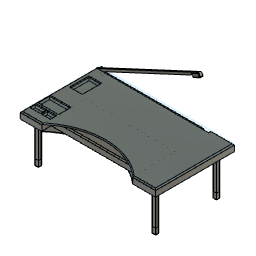
study pad (1) (Autodesk Fusion 360 design; units mm, degrees)
Autodesk Fusion 360 part; units mm, degrees
sketch "Sketch1" plane through (0, 0, 0) normal (0, 0, 1) x (1, 0, 0)
  line L0 (30, -17.5) -> (-30, -17.5)
  line L1 (-30, -17.5) -> (-30, 17.5)
  line L2 (-30, 17.5) -> (30, 17.5)
  line L3 (30, 17.5) -> (30, -17.5)
  line L4 (30, -17.5) -> (-30, 17.5) construction
  line L5 (-30, -17.5) -> (30, 17.5) construction
  dimension "d1" = 60
  dimension "d2" = 35
  constraint horizontal L0
  constraint perpendicular L0 L1
  constraint parallel L0 L2
  constraint parallel L1 L3
  constraint coincident L4 origin
  constraint coincident L5 origin
  measures "d1" distance of L1.end L2.end
  measures "d2" distance of L0.end L1.end
extrude "Extrude1" add sketch "Sketch1" along normal blind 3 makes body 1
sketch "Sketch2" plane through (0, 0, 3) normal (0, 0, 1) x (-1, 0, 0)
  line L0 (-30, -17.5) -> (30, -17.5)
  line L1 (30, -17.5) -> (30, 17.5)
  line L2 (30, 17.5) -> (-30, 17.5)
  line L3 (-30, 17.5) -> (-30, -17.5)
  arc A0 (-19.8527, 17.5) -> (20.3005, 17.5) centre (0.2239, 40.618) ccw
  line L4 (20.3005, 17.5) -> (-19.8527, 17.5)
  constraint coincident L2 A0.start
  constraint coincident L2 A0.end
extrude "Extrude2" cut sketch "Sketch2" against normal blind 6 contours L2 A0 L4 bodies 1
sketch "Sketch3" plane through (0, 17.5, 0) normal (0, 1, 0) x (-1, 0, 0)
  line L0 (-30, 0) -> (30, 0)
  line L1 (30, 0) -> (30, 3)
  line L2 (30, 3) -> (-30, 3)
  line L3 (-30, 3) -> (-30, 0)
  line L4 (20.3271, 2.6431, -39) -> (-19.8499, 2.6431, -39)
  line L5 (-19.8499, 2.6431, -39) -> (-19.8499, 0.2045, -39)
  line L6 (-19.8499, 0.2045, -39) -> (20.3271, 0.2045, -39)
  line L7 (20.3271, 0.2045, -39) -> (20.3271, 2.6431, -39)
sketch "Sketch4" plane through (0, 0, 0) normal (0, 1, 0) x (1, 0, 0)
extrude "Extrude3" cut sketch "Sketch3" along normal blind 23 contours L4 L5 L6 L7 in plane through (0, -21.5, 0) normal (0, 1, 0) bodies 1
sketch "Sketch5" plane through (0, 0, 3) normal (0, 0, 1) x (-1, 0, 0)
  arc A0 (-19.8527, 17.5) -> (20.3005, 17.5) centre (0.2239, 40.618) ccw
  line L0 (-19.8527, 17.5) -> (-30, 17.5)
  line L1 (-30, 17.5) -> (-30, -17.5)
  line L2 (-30, -17.5) -> (30, -17.5)
  line L3 (30, -17.5) -> (30, 17.5)
  line L4 (30, 17.5) -> (20.3005, 17.5)
sketch "Sketch6" plane through (0, 0, 0) normal (0, 0, 1) x (1, 0, 0)
sketch "Sketch7" plane through (0, 1.5, 0) normal (0, -1, 0) x (1, 0, 0)
  line L0 (-20.3271, 2.6431) -> (-20.3271, 0.2045)
  line L1 (-20.3271, 0.2045) -> (19.8499, 0.2045)
  line L2 (19.8499, 0.2045) -> (19.8499, 2.6431)
  line L3 (19.8499, 2.6431) -> (-20.3271, 2.6431)
  line L4 (-20.2486, -3.4362) -> (19.7746, -3.4362)
  line L5 (19.7746, -3.4362) -> (19.7746, -5.7391)
  line L6 (19.7746, -5.7391) -> (-20.2486, -5.7391)
  line L7 (-20.2486, -5.7391) -> (-20.2486, -3.4362)
  constraint horizontal L4
  constraint vertical L5
  constraint horizontal L6
  constraint vertical L7
sketch "Sketch8" plane through (0, 0, 0) normal (0, 1, 0) x (1, 0, 0)
extrude "Extrude4" add sketch "Sketch7" along normal blind 1 separate body contours L4 L5 L6 L7 makes body 2
sketch "Sketch9" plane through (0, 1.5, 0) normal (0, 1, 0) x (-1, 0, 0)
  line L0 (-19.7746, -5.7391) -> (20.2486, -5.7391)
  line L1 (20.2486, -5.7391) -> (20.2486, -3.4362)
  line L2 (20.2486, -3.4362) -> (-19.7746, -3.4362)
  line L3 (-19.7746, -3.4362) -> (-19.7746, -5.7391)
  line L4 (-19.7746, -4.5148) -> (20.2486, -4.5148)
  line L5 (20.2486, -4.5148) -> (20.2486, -5.7391)
  line L6 (20.2486, -5.7391) -> (-19.7746, -5.7391)
  line L7 (-19.7746, -5.7391) -> (-19.7746, -4.5148)
  constraint horizontal L4
  constraint vertical L5
  constraint horizontal L6
  constraint vertical L7
  constraint coincident L0.end L1.start
  constraint coincident L3 L4.start
extrude "Extrude5" add sketch "Sketch9" along normal blind 10 contours L0 L1 L3 L4 L5 L6 L7 bodies 2
move_body "Move1" bodies 2 to x (1, 0, 0) y (0, 1, 0) z (0, 0, 1) at (0, -21, 6)
move_body "Move2" bodies 2 to x (1, 0, 0) y (0, 1, 0) z (0, 0, 1) at (0, 9, 0)
move_body "Move3" bodies 2 to x (1, 0, 0) y (0, 1, 0) z (0, 0, 1) at (0, -2, 0)
sketch "Sketch10" plane through (0, 0, 3) normal (0, 0, 1) x (-1, 0, 0)
  line L0 (28, -11) -> (23, -11)
  line L1 (23, -11) -> (23, -3)
  line L2 (23, -3) -> (28, -3)
  line L3 (28, -3) -> (28, -11)
  dimension "d13" = 5
  dimension "d14" = 8
  constraint horizontal L0
  constraint vertical L1
  constraint horizontal L2
  constraint vertical L3
  measures "d13" distance of L0.start L0.end
  measures "d14" distance of L0.start L2.end
extrude "Extrude6" cut sketch "Sketch10" against normal blind 1.5 bodies 1
sketch "Sketch11" plane through (0, 0, 3) normal (0, 0, 1) x (1, 0, 0)
  line L0 (-29.5, -5) -> (-20.5, -5)
  line L1 (-20.5, -5) -> (-20.5, -10)
  line L2 (-20.5, -10) -> (-29.5, -10)
  line L3 (-29.5, -10) -> (-29.5, -5)
  line L4 (-29.5, -11.3721) -> (-25, -11.3721)
  line L5 (-25, -11.3721) -> (-25, -13.5948)
  line L6 (-25, -13.5948) -> (-29.5, -13.5948)
  line L7 (-29.5, -13.5948) -> (-29.5, -11.3721)
  line L8 (-20.5, -11.3721) -> (-24.054, -11.3721)
  line L9 (-24.054, -11.3721) -> (-24.054, -13.5948)
  line L10 (-24.054, -13.5948) -> (-20.5, -13.5948)
  line L11 (-20.5, -13.5948) -> (-20.5, -11.3721)
  constraint horizontal L0
  constraint vertical L1
  constraint horizontal L2
  constraint vertical L3
  constraint horizontal L4
  constraint vertical L5
  constraint horizontal L6
  constraint vertical L7
  constraint horizontal L8
  constraint vertical L9
  constraint horizontal L10
  constraint vertical L11
sketch "Sketch12" plane through (0, 0, 3) normal (0, 0, 1) x (1, 0, 0)
extrude "Extrude7" cut sketch "Sketch11" against normal blind 1.5 bodies 1
sketch "Sketch13" plane through (0, 0, 0) normal (0, 1, 0) x (1, 0, 0)
sketch "Sketch14" plane through (0, 0, 0) normal (0, 0, 1) x (1, 0, 0)
sketch "Sketch15" plane through (0, 0, 0) normal (0, 0, -1) x (1, 0, 0)
  arc A0 (-20.3005, 17.5) -> (19.8527, 17.5) centre (-0.2239, 40.618) ccw
  line L0 (-20.3005, 17.5) -> (-30, 17.5)
  line L1 (-30, 17.5) -> (-30, -17.5)
  line L2 (-30, -17.5) -> (30, -17.5)
  line L3 (30, -17.5) -> (30, 17.5)
  line L4 (30, 17.5) -> (19.8527, 17.5)
sketch "Sketch16" plane through (0, 0, 0) normal (0, 0, 1) x (1, 0, 0)
  line L0 (-34.64, -16.2701) -> (-33.3003, -16.2701)
  line L1 (-33.3003, -16.2701) -> (-33.3003, -17.4238)
  line L2 (-33.3003, -17.4238) -> (-34.64, -17.4238)
  line L3 (-34.64, -17.4238) -> (-34.64, -16.2701)
  line L4 (-34.5712, -16.347) -> (-33.3606, -16.347)
  line L5 (-33.3606, -16.347) -> (-33.3606, -17.3584)
  line L6 (-33.3606, -17.3584) -> (-34.5712, -17.3584)
  line L7 (-34.5712, -17.3584) -> (-34.5712, -16.347)
  line L8 (-36.4, -16.2) -> (-34.95, -16.2)
  line L9 (-34.95, -16.2) -> (-34.95, -17.5)
  line L10 (-34.95, -17.5) -> (-36.4, -17.5)
  line L11 (-36.4, -17.5) -> (-36.4, -16.2)
  line L12 (-36.4634, -16.1288) -> (-34.8788, -16.1288)
  line L13 (-34.8788, -16.1288) -> (-34.8788, -17.5639)
  line L14 (-34.8788, -17.5639) -> (-36.4634, -17.5639)
  line L15 (-36.4634, -17.5639) -> (-36.4634, -16.1288)
  constraint horizontal L0
  constraint vertical L1
  constraint horizontal L2
  constraint vertical L3
  constraint horizontal L4
  constraint vertical L5
  constraint horizontal L6
  constraint vertical L7
  constraint horizontal L8
  constraint vertical L9
  constraint horizontal L10
  constraint vertical L11
  constraint horizontal L12
  constraint vertical L13
  constraint horizontal L14
  constraint vertical L15
extrude "Extrude8" add sketch "Sketch16" along normal blind 16 separate body makes body 3 at (-35.9352, -16.1288, 10.6667) makes body 4 at (-34.1934, -16.2701, 5.3333)
move_body "Move4" bodies 4 to x (1, 0, 0) y (0, 1, 0) z (0, 0, 1) at (-1.7, 0, 0)
move_body "Move5" bodies 4 to x (1, 0, 0) y (0, 1, 0) z (0, 0, 1) at (0, 0, 14)
sketch "Sketch17" plane through (0, 0, 30) normal (0, 0, 1) x (-1, 0, 0)
  line L0 (35.0606, 17.3584) -> (36.2712, 17.3584)
  line L1 (36.2712, 17.3584) -> (36.2712, 16.347)
  line L2 (36.2712, 16.347) -> (35.0606, 16.347)
  line L3 (35.0606, 16.347) -> (35.0606, 17.3584)
  line L4 (36.34, 17.4238) -> (35.0003, 17.4238)
  line L5 (35.0003, 17.4238) -> (35.0003, 16.2701)
  line L6 (35.0003, 16.2701) -> (36.34, 16.2701)
  line L7 (36.34, 16.2701) -> (36.34, 17.4238)
  line L8 (36.5, 16.1) -> (34.8456, 16.1)
  line L9 (34.8456, 16.1) -> (34.8456, 17.5928)
  line L10 (34.8456, 17.5928) -> (36.5, 17.5928)
  line L11 (36.5, 17.5928) -> (36.5, 16.1)
  constraint horizontal L8
  constraint vertical L9
  constraint horizontal L10
  constraint vertical L11
extrude "Extrude9" add sketch "Sketch17" along normal blind 0.1 contours L0 L1 L2 L3 | L4 L5 L6 L7 | L8 L9 L10 L11 bodies 4
move_body "Move6" bodies 3 to x (1, 0, 0) y (0, 1, 0) z (0, 0, 1) at (0, 0, 11.5)
move_body "Move7" bodies 3 4 to x (1, 0, 0) y (0, 1, 0) z (0, 0, 1) at (1, 0, -30)
copy_body "CopyPasteBodies1" bodies 4 3 makes body 5 makes body 6
move_body "Move8" bodies 5 6 to x (1, 0, 0) y (0, 1, 0) z (0, 0, 1) at (60, 4, 0)
copy_body "CopyPasteBodies2" bodies 4 3 makes body 7 makes body 8
move_body "Move9" bodies 7 8 to x (1, 0, 0) y (0, 1, 0) z (0, 0, 1) at (8, 31, 0)
copy_body "CopyPasteBodies3" bodies 4 3 makes body 9 makes body 10
move_body "Move10" bodies 9 10 to x (1, 0, 0) y (0, 1, 0) z (0, 0, 1) at (60, 31, 0)
move_body "Move11" bodies 4 3 to x (1, 0, 0) y (0, 1, 0) z (0, 0, 1) at (8, 4, 0)
sketch "Sketch18" plane through (0, 0, 3) normal (0, 0, 1) x (-1, 0, 0)
sketch "Sketch19" plane through (0, 17.5, 0) normal (0, 1, 0) x (-1, 0, 0)
  line L0 (-30, 0) -> (30, 0)
  line L1 (30, 0) -> (30, 3)
  line L2 (30, 3) -> (-30, 3)
  line L3 (-30, 3) -> (-30, 0)
sketch "Sketch20" plane through (0, 0, 3) normal (0, 0, 1) x (-1, 0, 0)
  line L0 (30, -17.5) -> (-20, -17.5)
  line L1 (-20, -17.5) -> (-20, -16)
  line L2 (-20, -16) -> (30, -16)
  line L3 (30, -16) -> (30, -17.5)
  constraint horizontal L0
  constraint vertical L1
  constraint horizontal L2
  constraint vertical L3
extrude "Extrude10" cut sketch "Sketch20" against normal blind 1 bodies 1
sketch "Sketch21" plane through (0, 17.5, 0) normal (0, 1, 0) x (-1, 0, 0)
sketch "Sketch22" plane through (0, 17.5, 0) normal (0, 1, 0) x (-1, 0, 0)
  line L0 (-20, 3) -> (-16.5, 3)
  line L1 (-16.5, 3) -> (-16.5, 1)
  line L2 (-16.5, 1) -> (-20, 1)
  line L3 (-20, 1) -> (-20, 3)
  constraint horizontal L0
  constraint vertical L1
  constraint horizontal L2
  constraint vertical L3
extrude "Extrude11" cut sketch "Sketch22" against normal blind 1.5 bodies 1
sketch "Sketch23" plane through (0, 17.5, 0) normal (0, 1, 0) x (-1, 0, 0)
  line L0 (-20, 3) -> (-20, 1)
  line L1 (-20, 1) -> (-16.5, 1)
  line L2 (-16.5, 1) -> (-16.5, 2)
  line L3 (-16.5, 2) -> (30, 2)
  line L4 (30, 2) -> (30, 3)
  line L5 (30, 3) -> (-20, 3)
  constraint vertical L0
  constraint perpendicular L0 L1
  constraint perpendicular L1 L2
  constraint perpendicular L2 L3
  constraint perpendicular L3 L4
  constraint perpendicular L0 L5
extrude "Extrude12" add sketch "Sketch23" against normal blind 1.5 separate body makes body 11
move_body "Move12" bodies 11 to x (0.906308, 0, 0.422618) y (0, 1, 0) z (-0.422618, 0, 0.906308) at (-1.4992, 0, 12.7246)
move_body "Move13" bodies 11 to x (1, 0, 0) y (0, 1, 0) z (0, 0, 1) at (0, 0, 1.5)
fillet "Fillet1" radius 0.8 1 edges at (-29.5337, 16.75, 3.3587) on bodies 11
move_body "Move14" bodies 11 to x (1, 0, 0) y (0, 1, 0) z (0, 0, 1) at (-0.05, 0, -1.6)
hole "Hole1" at (-29.2581, 17.5, 2.4428) direction (0, -1, 0) diameter 0.5 depth 2.6 tip angle 118 bodies 1 11
sketch "Sketch24" plane through (0, 17.5, 0) normal (0, 1, 0) x (-1, 0, 0)
hole "Hole2" at (-27.2077, 16, 2.4392) direction (0, -1, 0) diameter 0.6 depth 0.9 tip angle 118 bodies 1
hole "Hole3" at (-25.8093, 16, 2.4533) direction (0, -1, 0) diameter 0.6 depth 1.3 tip angle 118 bodies 1
sketch "Sketch25" plane through (0, 0, 0) normal (0, 1, 0) x (1, 0, 0)
  circle A0 centre (-30.5589, -2.4419) radius 0.2002
sketch "Sketch26" plane through (0, 17.5, 0) normal (0, 1, 0) x (-1, 0, 0)
extrude "Extrude13" add sketch "Sketch25" along normal blind 1 separate body makes body 12
move_body "Move15" bodies 12 to x (1, 0, 0) y (0, 1, 0) z (0, 0, 1) at (0, 16.8, 0)
extrude "Extrude14" add 1 faces at (-30.68, 16.8, 2.3944) along direction (0, -1, 0) blind 1.2 on bodies 12 bodies 12
sketch "Sketch27" plane through (0, 17.8, 0) normal (0, 1, 0) x (-1, 0, 0)
  circle A0 centre (30.5589, 2.4419) radius 0.2002
  circle A1 centre (30.5589, 2.4419) radius 0.3775
  constraint concentric A0 A1
extrude "Extrude15" add sketch "Sketch27" along normal blind 0.3 contours A0 | A1 bodies 12
fillet "Fillet2" radius 0.175 1 edges at (-30.2069, 18.1, 2.3054) on bodies 12
copy_body "CopyPasteBodies4" bodies 12 makes body 13
move_body "Move16" bodies 13 to x (1, 0, 0) y (0, 1, 0) z (0, 0, 1) at (1.3, 0, 0)
move_body "Move17" bodies 12 to x (1, 0, 0) y (0, 1, 0) z (0, 0, 1) at (3.3, 0, 0)
fillet "Fillet3" radius 0.3 16 edges at (-25, -10, 3) (-29.5, -7.5, 3) (-25, -5, 3) (-20.5, -7.5, 3) (-22.277, -11.3721, 3) (-20.5, -12.4834, 3) (-22.277, -13.5948, 3) (-24.054, -12.4834, 3) (-25, -12.4834, 3) (-27.25, -11.3721, 3) (-27.25, -13.5948, 3) (-29.5, -12.4834, 3) (-25.5, 11, 3) (-23, 7, 3) (-28, 7, 3) (-25.5, 3, 3) on bodies 1
chamfer "Chamfer1" distance 0.5 angle 45 7 edges at (-7.3486, 17.5, 13.2304) (30, 0, 3) (25, 17.5, 3) (24.9263, -17.5, 3) (-0.2239, -9.9992, 3) (-25.1502, -17.5, 3) (-30, -0.75, 3) on bodies 1 11
sketch "Sketch28" plane through (0, 16, 0) normal (0, -1, 0) x (1, 0, 0)
  circle A0 centre (-29.2581, 2.4428) radius 0.25
  arc A1 (-29.9218, 2.4837) -> (-28.8587, 2.0968) centre (-29.1968, 2.8218) ccw
  line L0 (-28.8587, 2.0968) -> (12.5596, 21.4104)
  line L1 (12.5596, 21.4104) -> (12.9822, 20.5041)
  line L2 (12.9822, 20.5041) -> (16.1543, 21.9833)
  line L3 (16.1543, 21.9833) -> (15.3091, 23.7959)
  line L4 (15.3091, 23.7959) -> (-30.0063, 2.665)
  line L5 (-30.0063, 2.665) -> (-29.9218, 2.4837)
  line L6 (12.3375, 21.8868) -> (12.9822, 20.5041)
  line L7 (16.1543, 21.9833) -> (15.4814, 23.4264)
  line L8 (12.3375, 21.8868) -> (15.4814, 23.4264)
  constraint coincident L1.end L2.start
  constraint perpendicular L2 L6
  constraint coincident L2.end L3.start
  constraint coincident L3 L7.end
  constraint perpendicular L2 L7
extrude "Extrude16" cut sketch "Sketch28" against normal blind 0.1 contours L1 L2 L3 L6 L7 L8 bodies 11
fillet "Fillet4" radius 0.25 7 edges at (14.5682, 16.1, 21.2437) (15.8178, 16.1, 22.7048) (16.1543, 16.8, 21.9833) (14.5682, 17.5, 21.2437) (12.9822, 16.8, 20.5041) (12.7709, 16.1, 20.9573) (12.7709, 17.5, 20.9573) on bodies 11
fillet "Fillet5" radius 0.85 2 edges at (-6.7596, 17.5, 12.9534) (-7.3486, 17, 13.2304) on bodies 11
sketch "Sketch29" plane through (0, 0, 0) normal (0, 0, -1) x (1, 0, 0)
  line L0 (-26.5, 11) -> (-14, 1)
  line L1 (-25, 12) -> (-13.0292, 2.4233)
  line L2 (-13.0292, 2.4233) -> (-14, 1)
  line L3 (-25, 12) -> (-26.5, 11)
  line L4 (-26, -12) -> (-13, -3)
  line L5 (-25, -13.5) -> (-11.8573, -4.5696)
  line L6 (-11.8573, -4.5696) -> (-13, -3)
  line L7 (-26, -12) -> (-25, -13.5)
  line L8 (23, 12) -> (24.0716, 10.4229)
  line L9 (24.0716, 10.4229) -> (13.3297, 3.1238)
  line L10 (13.3297, 3.1238) -> (12.17, 4.8305)
  line L11 (12.17, 4.8305) -> (23, 12)
  line L12 (24, -12) -> (14, -4)
  line L13 (14, -4) -> (13.0328, -5.2091)
  line L14 (13.0328, -5.2091) -> (23.0575, -13.2288)
  line L15 (23.0575, -13.2288) -> (24, -12)
  constraint parallel L0 L1
  constraint perpendicular L5 L8
  constraint perpendicular L8 L9
  constraint perpendicular L5 L10
  constraint perpendicular L12 L13
  constraint perpendicular L13 L14
extrude "Extrude17" cut sketch "Sketch29" against normal blind 0.1 bodies 1
